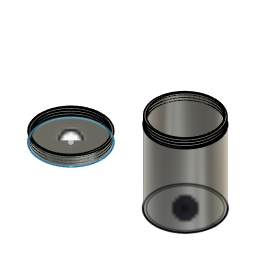
tea_container v4 (Autodesk Fusion 360 design; units mm, degrees)
Autodesk Fusion 360 part; units mm, degrees
sketch "草图1" plane through (0, 0, 0) normal (0, 0, 1) x (1, 0, 0)
  circle A0 centre (0, 0) radius 37.5
  circle A1 centre (0, 0) radius 38
  circle A2 centre (0, 0) radius 35
  dimension "d1" = 75
  dimension "d2" = 76
  dimension "d20" = 70
  constraint coincident A0.centre A1.centre
  constraint concentric A0 A1
  measures "d1" diameter of A0
  measures "d2" diameter of A1
  measures "d20" diameter of A2
extrude "拉伸10" add sketch "草图1" along normal blind 2 contours A2 makes body 1
extrude "拉伸11" add sketch "草图1" along normal blind 102 contours A0 bodies 1
extrude "拉伸12" add sketch "草图1" along normal blind 92 contours A1 bodies 1
thread "螺纹7" "ISO Metric profile 75.0 M75x3 6g" major diameter 74.7645 minor diameter 71.3239 pitch 3 angle 60 modelled right hand crest width 0.422 on face at (37.3137, -3.7338, 95.3333) crest through (37.3822, 0, 91.25) on bodies 1
sketch "草图2" plane through (0, 0, 0) normal (0, 0, 1) x (1, 0, 0)
  circle A0 centre (-145.2795, 0.1934) radius 37.5
  circle A1 centre (-145.2795, 0.1934) radius 38.5
  dimension "d56" = 75
  dimension "d57" = 77
  constraint concentric A0 A1
  measures "d56" diameter of A0
  measures "d57" diameter of A1
extrude "拉伸17" add sketch "草图2" along normal blind 12 separate body makes body 2
extrude "拉伸18" add sketch "草图2" along normal blind 2 contours A0 bodies 2
thread "螺纹10" "ISO Metric profile 75.0 M75x3 6H" major diameter 75.3564 minor diameter 72.0024 pitch 3 angle 60 modelled right hand crest width 0.8135 on face at (-107.9659, -3.5403, 8.6667) crest through (-109.2783, 0.1934, 2.75) on bodies 2
